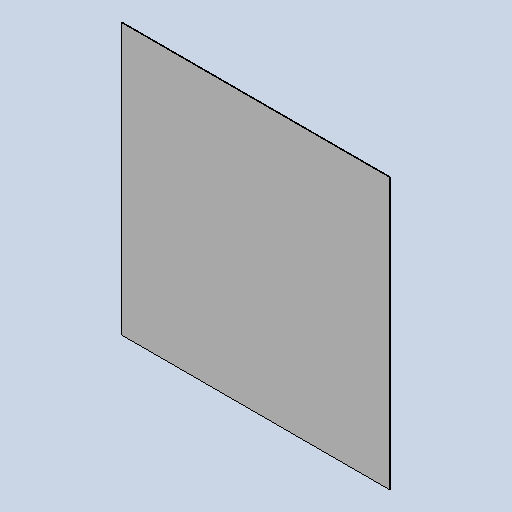
# Autodesk Inventor part: GBK 1111 shield 1
Saved by Autodesk Inventor 2026.2 (Build 302298010, 298A)
## iProperties
Created: 2026-04-17
Part Number: GBK 1111 shield 1
Material: Steel
Document SubType Name: Sheet Metal
Designer: admin
Density: 7.85 g/cm^3
Sheet Metal Rule: Default_mm
Appearance: Default
Mass: 69243.3 g
Surface Area: 44341.6 cm^2
Volume: 8820.8 cm^3
Flat Pattern Width: 148 cm
Flat Pattern Length: 149 cm
Flat Pattern Area: 22052 cm^2
Sheet Metal Width: 1480,000 mm
Sheet Metal Length: 1490,000 mm
Sheet Metal Area: 2205200,000 mm^2
Stock Number: 1115
Author: admin
Autodesk Inventor part; units mm, degrees
ref_plane "YZ Plane" through (0, 0, 0) normal (1, 0, 0) x (0, 1, 0)
ref_plane "XZ Plane" through (0, 0, 0) normal (0, 1, 0) x (-1, 0, 0)
ref_plane "XY Plane" through (0, 0, 0) normal (0, 0, 1) x (1, 0, 0)
sketch "Sketch1" plane through (0, 0, 0) normal (0, 0, 1) x (1, 0, 0)
  line L0 (740, -745) -> (-740, -745)
  line L1 (-740, -745) -> (-740, 745)
  line L2 (-740, 745) -> (740, 745)
  line L3 (740, 745) -> (740, -745)
  line L4 (740, -745) -> (-740, 745) construction
  line L5 (-740, -745) -> (740, 745) construction
  point P0 (0, 0)
  dimension "d0" = 1480
  dimension "d1" = 1490
  measures "d0" distance of L1.end L2.end
  measures "d1" distance of L0.end L1.end
extrude "Plate1" add sketch "Sketch1" along normal blind 4
sketch "Sketch3" plane through (0, 0, 0) normal (0, 0, -1) x (-1, 0, 0)
  line L0 (488.1353, -557.3462) -> (488.1353, -1055.4823) construction
  line L1 (488.1353, -1055.4823) -> (448.5081, -1055.4823) construction
  line L2 (448.5081, -1055.4823) -> (448.5081, -557.3462) construction
  line L3 (448.5081, -557.3462) -> (488.1353, -557.3462) construction
  line L4 (710, -489.5) -> (770, -489.5)
  line L5 (710, -489.5) -> (710, -485.5)
  line L6 (710, 7.1667) -> (770, 7.1667)
  line L7 (710, 7.1667) -> (710, 11.1667)
  line L8 (710, 503.8333) -> (770, 503.8333)
  line L9 (710, 503.8333) -> (710, 507.8333)
  line L10 (-738.6395, -489.5) -> (-680, -489.5)
  line L11 (-680, -489.5) -> (-680, -485.5)
  line L12 (-738.6395, 7.1667) -> (-680, 7.1667)
  line L13 (-680, 7.1667) -> (-680, 11.1667)
  line L14 (-738.6395, 503.8333) -> (-680, 503.8333)
  line L15 (-680, 503.8333) -> (-680, 507.8333)
  line L16 (-330.3944, -493) -> (-330.3944, -590)
  line L17 (-330.3944, -590) -> (-334.3934, -590)
  line L18 (169.7342, -493) -> (169.7342, -590)
  line L19 (169.7342, -590) -> (165.7352, -590)
  line L20 (669.8628, -493) -> (669.8628, -590)
  line L21 (669.8628, -590) -> (665.8638, -590)
  ellipse E0 centre (669.8628, 745) end of major axis (669.8628, 775) minor radius 0.6803 (669.8628, 715) -> (669.8628, 775) ccw
  line L22 (669.8628, 715) -> (665.8638, 715)
  ellipse E1 centre (169.7342, 745) end of major axis (169.7342, 775) minor radius 0.6803 (169.7342, 715) -> (169.7342, 775) ccw
  line L23 (169.7342, 715) -> (165.7352, 715)
  ellipse E2 centre (-330.3944, 745) end of major axis (-330.3944, 775) minor radius 0.6803 (-330.3944, 715) -> (-330.3944, 775) ccw
  line L24 (-330.3944, 715) -> (-334.3934, 715)
  constraints: 42 end point, 12 horizontal, 9 vertical, 53 other
mark "Mark2"
equation "\"d0\" = Лист_ширина"
equation "\"d1\" = 0.5 * Лист_длина"
equation "\"d2\" = Thickness"
equation "\"BendRadius\" = Thickness"
equation "\"BendReliefWidth\" = Thickness"
equation "\"BendReliefDepth\" = 0.5 * Thickness"
equation "\"CornerReliefSize\" = 4 * Thickness"
equation "\"MinimumRemnant\" = 2 * Thickness"
equation "\"TransitionRadius\" = BendRadius"
equation "\"JacobiRadiusSize\" = BendRadius"
equation "\"GapSize\" = Thickness"
equation "\"Лист_ширина\" = 1480"
equation "\"Лист_длина\" = 2980"
equation "\"Thickness\" = 4"
body "Solid1"
